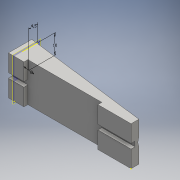
# Autodesk Inventor part: support_lcd_v2
Saved by Autodesk Inventor 2016 (Build 200138000, 138)
## iProperties
Created: 2019-02-19
Part Number: support_lcd_v2
Material: Generic
Document SubType Name: Modeling
Designer: mbouhier
Density: 1 g/cm^3
Appearance: Default
Author: mbouhier
Autodesk Inventor part; units mm, degrees
ref_plane "YZ Plane" through (0, 0, 0) normal (1, 0, 0) x (0, 1, 0)
ref_plane "XZ Plane" through (0, 0, 0) normal (0, 1, 0) x (-1, 0, 0)
ref_plane "XY Plane" through (0, 0, 0) normal (0, 0, 1) x (1, 0, 0)
sketch "Sketch1" plane through (0, 0, 0) normal (0, 0, 1) x (1, 0, 0)
  line L0 (0, 0) -> (0, 4)
  line L1 (0, 0) -> (-63, 0)
  line L2 (-63, 0) -> (-63, 12)
  line L3 (-63, 12) -> (0, 4)
  dimension "d0" = 4
  dimension "d1" = 63
  dimension "d2" = 12
  constraints: 8 end point, 1 horizontal, 1 perpendicular, 1 vertical
  measures "d0" distance of L0.start L0.end
  measures "d1" distance of L0.start L1.end
  measures "d2" distance of L1.end L2.end
extrude "Extrusion1" add sketch "Sketch1" along normal blind 20
sketch "Sketch2" plane through (-63, 0, 0) normal (-1, 0, 0) x (0, 0, 1)
  line L0 (0, 0) -> (20, 0) projected
  line L1 (10, 0) -> (8.75, 0)
  line L2 (8.75, 0) -> (8.75, 2)
  line L3 (8.75, 2) -> (10, 2)
  line L4 (10, 2) -> (10, 0)
  line L5 (10, 0) -> (11.25, 0)
  line L6 (11.25, 0) -> (11.25, 2)
  line L7 (11.25, 2) -> (10, 2)
  line L8 (10, 2) -> (10, 0)
  line L9 (0, 0) -> (20, 0) projected
  dimension "d5" = 1.25
  dimension "d6" = 2
  dimension "d7" = 1.25
  constraints: 16 end point, 4 parallel, 2 horizontal, 2 midpoint, 2 perpendicular, 1 point on line
  measures "d5" distance of L2.end L3.end
  measures "d6" distance of L1.end L2.end
  measures "d7" distance of L7.end L6.end
extrude "Extrusion2" cut sketch "Sketch2" against normal through all
ref_plane "Work Plane1" through (-60, 0, 0) normal (-1, 0, 0) x (0, 0, 1)
sketch "Sketch3" plane through (-60, 0, 0) normal (-1, 0, 0) x (0, 0, 1)
  line L0 (0, 12) -> (20, 12) projected
  circle A0 centre (10, 7.5) radius 4
  line L1 (6, 7.5) -> (14, 7.5)
  line L2 (14, 7.5) -> (14, 12)
  line L3 (14, 12) -> (6, 12)
  line L4 (6, 12) -> (6, 7.5)
  line L5 (20, 4) -> (20, 12) projected
  point P0 (0, 0)
  dimension "d12" = 8
  dimension "d11" = 4.5
  dimension "d27" = 10
  constraints: 8 end point, 2 parallel, 1 coincident, 1 horizontal, 1 horizontal alignment, 1 perpendicular, 1 point on line, 2 other
  measures "d11" distance from line of L0 point (10, 7.5)
  measures "d27" distance from line of point (10, 7.5) L5
extrude "Extrusion3" cut sketch "Sketch3" against normal through all
hole "Hole1" at (-60, 7.5, 10) direction (-1, 0, 0) diameter 4.5 end through all
sketch "Sketch4" plane through (-63, 0, 0) normal (0, -1, 0) x (1, 0, 0)
  point P0 (63, 0)
sketch "Sketch5" plane through (-63, 0, 0) normal (0, -1, 0) x (1, 0, 0)
  line L0 (46, 20) -> (46, 0)
  line L1 (8, 0) -> (46, 0)
  line L2 (46, 0) -> (46, 20)
  line L3 (46, 20) -> (8, 20)
  line L4 (8, 20) -> (8, 0)
  point P0 (0, 0)
  dimension "d23" = 46
  dimension "d26" = 8
  constraints: 10 end point, 2 parallel, 1 horizontal, 1 perpendicular
  measures "d23" distance of L0.end point (0, 0)
  measures "d26" distance of L1.start point (0, 0)
extrude "Extrusion4" cut sketch "Sketch5" against normal up to surface (2 mm away)
body "Solid1"
